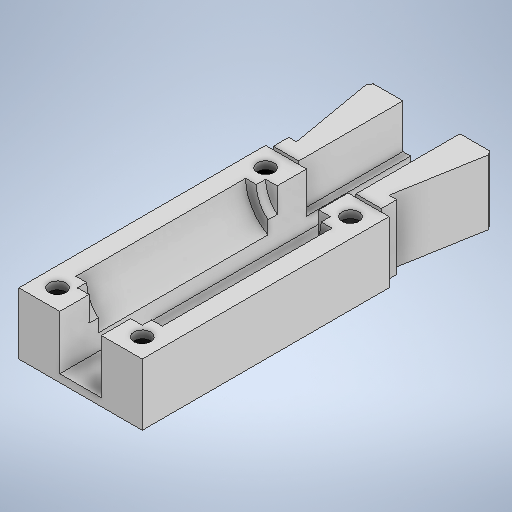
# Autodesk Inventor part: SwitchLeverUnit_LowerCase
Saved by Autodesk Inventor 2025.1 (Build 291241000, 241)
## iProperties
Created: 2025-03-08
Part Number: SwitchLeverUnit_LowerCase
Material: 一般
Document SubType Name: Modeling
Designer: kumagai
Density: 1 g/cm^3
Appearance: 既定
d0: 8.400 mm
d1: 5.400 mm
d2: 7.000 mm
d3: 4.000 mm
d4: 16.000 mm
d5: 32.000 mm
d6: 11.200 mm
d7: 8.000 mm
d8: 0.00 deg
d10: 0.00 deg
d11: 22.000 mm
d12: 0.00 deg
d13: 24.400 mm
d14: 0.00 deg
d15: 3.300 mm
d16: 2.200 mm
d17: 2.500 mm
d18: 2.500 mm
d20: 0.00 deg
d21: 7.000 mm
d23: 16.000 mm
d24: 12.000 mm
d25: 14.000 mm
d26: 2.000 mm
d28: 11.500 mm
d29: 7.400 mm
d30: 8.400 mm
d32: 5.700 mm
d34: 0.500 mm
d37: 6.750 mm
Author: kumagai
Autodesk Inventor part; units mm, degrees
ref_plane "YZ Plane" through (0, 0, 0) normal (1, 0, 0) x (0, 1, 0)
ref_plane "XZ Plane" through (0, 0, 0) normal (0, 1, 0) x (-1, 0, 0)
ref_plane "XY Plane" through (0, 0, 0) normal (0, 0, 1) x (1, 0, 0)
sketch "DrumSketch" plane through (0, 0, 0) normal (0, 0, 1) x (1, 0, 0)
  line L0 (0, 8.12) -> (0, -9.52) projected
  line L1 (-7.84, 0) -> (7.84, 0) projected
  circle A0 centre (0, 0) radius 4.2
  line L2 (-2.7, -3) -> (2.7, -3)
  line L3 (2.7, 0) -> (2.7, -7)
  line L4 (2.7, -7) -> (-2.7, -7)
  line L5 (-2.7, -7) -> (-2.7, 0)
  circle A1 centre (0, 0) radius 5.6
  dimension "d0" = 8.4
  dimension "d1" = 5.4
  dimension "d2" = 7
  dimension "d3" = 4
  dimension "d6" = 11.2
  constraints: 8 end point, 4 point on line, 2 centre point, 2 coincident, 1 other
  measures "d0" diameter of A0
  measures "d1" distance between parallel lines of L3 L5
  measures "d2" distance between parallel lines of L4 L1
  measures "d3" distance between parallel lines of L4 L2
  measures "d6" diameter of A1
sketch "BodySketch" plane through (0, 0, 0) normal (0, 1, 0) x (-1, 0, 0)
  line L0 (8, 16) -> (-8, 16)
  line L1 (-8, 16) -> (-8, -16)
  line L2 (-8, -16) -> (8, -16)
  line L3 (8, -16) -> (8, 16)
  line L4 (0, -38.6) -> (0, 25.1) projected
  line L5 (-11.2, 0) -> (11.2, 0) projected
  circle A0 centre (5.5, 13.5) radius 1.1
  circle A1 centre (5.5, 13.5) radius 1.65
  circle A2 centre (5.5, -13.5) radius 1.1
  circle A3 centre (5.5, -13.5) radius 1.65
  circle A4 centre (-5.5, 13.5) radius 1.1
  circle A5 centre (-5.5, 13.5) radius 1.65
  circle A6 centre (-5.5, -13.5) radius 1.65
  circle A7 centre (-5.5, -13.5) radius 1.1
  line L6 (7, -16) -> (7, -18)
  line L7 (7, -18) -> (6, -18)
  line L8 (6, -18) -> (8, -29.5)
  line L9 (8, -29.5) -> (-8, -29.5)
  line L10 (-8, -29.5) -> (-6, -18)
  line L11 (-6, -18) -> (-7, -18)
  line L12 (-7, -18) -> (-7, -16)
  line L13 (3.7, -29.5) -> (3.7, -16)
  line L14 (-3.7, -29.5) -> (-3.7, -16)
  line L15 (2.4888, -22.75) -> (1.2404, -22.75)
  circle A8 centre (5.5, 13.5) radius 1.75
  circle A9 centre (5.5, -13.5) radius 1.75
  circle A10 centre (-5.5, 13.5) radius 1.75
  circle A11 centre (-5.5, -13.5) radius 1.75
  point P0 (0, 0)
  point P1 (-8, 0)
  point P2 (0, 16)
  point P3 (8, 0)
  point P4 (0, -16)
  dimension "d4" = 16
  dimension "d5" = 32
  dimension "d15" = 3.3
  dimension "d16" = 2.2
  dimension "d17" = 2.5
  dimension "d18" = 2.5
  dimension "d23" = 16
  dimension "d24" = 12
  dimension "d25" = 14
  dimension "d26" = 2
  dimension "d28" = 11.5
  dimension "d29" = 7.4
  dimension "d37" = 6.75
  dimension "d38" = 6.75
  dimension "d39" = 22.75
  dimension "d40" = 3.5
  constraints: 28 end point, 12 centre point, 12 symmetric about line, 7 point on line, 5 coincident, 1 horizontal, 1 vertical, 12 other
  measures "d4" distance between parallel lines of L1 L3
  measures "d5" distance between parallel lines of L2 L0
  measures "d15" diameter of A1
  measures "d16" diameter of A0
  measures "d17" distance from line of L3 A0.centre
  measures "d18" distance from line of L0 A0.centre
  measures "d23" distance of L9.end L8.end
  measures "d24" distance of L10.end L7.end
  measures "d25" distance between parallel lines of L12 L6
  measures "d26" distance between parallel lines of L2 L7
  measures "d28" distance between parallel lines of L11 L9
  measures "d29" distance between parallel lines of L14 L13
  measures "d37" distance between parallel lines of L9 L15
  measures "d38" distance between parallel lines of L15 L2
  measures "d39" distance between parallel lines of L5 L15
  measures "d40" diameter of A8
extrude "MainBody" add sketch "BodySketch" against normal blind 8 contours L3 L5 L4 L0 | L4 L5 L1 L0 | L3 L2 L4 L5 | L4 L2 L1 L5 | A0 | A1 | A2 | A3 | A4 | A5 | A6 | A7 | A8 | A9 | A10 | A11
extrude "TrapConnector" add sketch "BodySketch" along normal blind 8.4 from surface at -8 contours L4 L9 L14 L2 | L2 L13 L9 L4 | L6 L7 L8 L9 L13 L2 | L14 L9 L10 L11 L12 L2
extrude "SliderChannel" cut sketch "DrumSketch" along normal through all both and the other way through all contours L1 L3 L2 L0 | L0 L2 L5 L1 | A1 L0 A0 L3 | L3 L4 L0 A1 | A1 L0 L4 L5 | L5 A0 L0 A1 | L2 L3 A0 L0 | L0 A0 L5 L2
extrude "TrapChannel" cut sketch "BodySketch" against normal blind 5.7 from surface at 0.4 contours L4 L9 L14 L2 | L2 L13 L9 L4
extrude "DrumChannel" cut sketch "DrumSketch" along normal mid plane 22 contours A1 L1 A0 L0 | L0 A0 L1 A1 | A0 L1 L0 | L0 L1 A0 | A1 L3 A0 L1 | L1 A0 L5 A1 | L1 L3 L2 L0 | L0 L2 L5 L1 | A0 L3 L1 | L1 L5 A0 | A1 L0 A0 L3 | L5 A0 L0 A1 | L2 L3 A0 L0 | L0 A0 L5 L2
extrude "DrumBearing" cut sketch "DrumSketch" along normal mid plane 24.4 contours A0 L1 L0 | L0 L1 A0 | L1 L3 L2 L0 | L0 L2 L5 L1 | A0 L3 L1 | L1 L5 A0 | L2 L3 A0 L0 | L0 A0 L5 L2
extrude "FixHoleTop" cut sketch "BodySketch" against normal through all contours A0 | A2 | A4 | A7
extrude "FixHoleMid" cut sketch "BodySketch" along normal blind 7 from surface at -8 contours A0 | A1 | A2 | A3 | A4 | A5 | A6 | A7
extrude "FixHoleBottom" cut sketch "BodySketch" along normal blind 4 from surface at -8 contours A0 | A1 | A2 | A3 | A4 | A5 | A6 | A7 | A8 | A9 | A10 | A11
chamfer "TrapEdgeChamfer" distance 0.5 angle 45 2 edges at (-8, -3.8, -29.5) (8, -3.8, -29.5)
equation "\"d23\" = LeverConnectTrapWidthBottom"
equation "\"d24\" = LeverConnectTrapWidthTop"
equation "\"d28\" = LeverConnectTrapDepth"
equation "\"d37\" = d38"
equation "\"d30\" = RailHeight"
equation "\"RHtmp\" = 8.4"
equation "\"RTtmp\" = 2"
equation "\"LeverConnectTrapWidthBottom\" = 16"
equation "\"LeverConnectTrapWidthTop\" = 12"
equation "\"LeverConnectTrapDepth\" = 11.5"
equation "\"RailHeight\" = 8.4"
